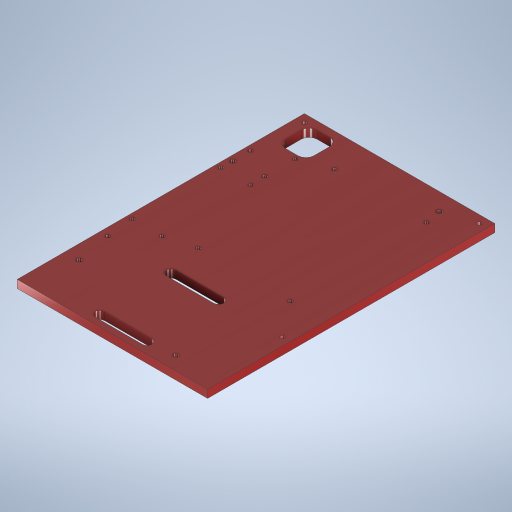
# Autodesk Inventor part: tamiya_chassis
Saved by Autodesk Inventor 2024 (Build 280153000, 153)
## iProperties
Created: 2024-01-24
Part Number: tamiya_chassis
Material: Generic
Document SubType Name: Modeling
Designer: critt
Density: 1 g/cm^3
Appearance: Default
Author: critt
## iProperties of the stored document tamiya_chassis_3DPrint.ipt
Created: 2024-01-26
Part Number: tamiya_chassis_3DPrint
Material: Generic
Document SubType Name: Modeling
Designer: critt
Density: 1 g/cm^3
Appearance: Default
Author: critt
Autodesk Inventor part; units mm, degrees
ref_plane "YZ Plane" through (0, 0, 0) normal (1, 0, 0) x (0, 1, 0)
ref_plane "XZ Plane" through (0, 0, 0) normal (0, 1, 0) x (-1, 0, 0)
ref_plane "XY Plane" through (0, 0, 0) normal (0, 0, 1) x (1, 0, 0)
sketch "Sketch1" plane through (0, 0, 0) normal (0, 1, 0) x (-1, 0, 0)
  line L0 (35.3225, -111.2173) -> (35.3225, -99.2173)
  arc A0 (39.3225, -95.2173) -> (35.3225, -99.2173) centre (39.3225, -99.2173) ccw
  line L1 (39.3225, -95.2173) -> (50.3225, -95.2173)
  line L2 (50.3225, -95.2173) -> (50.3225, -19.2173)
  line L3 (50.3225, -19.2173) -> (41.3225, -10.2173)
  line L4 (41.3225, -10.2173) -> (41.3225, 19.7827)
  line L5 (41.3225, 19.7827) -> (50.3225, 29.7827)
  line L6 (50.3225, 29.7827) -> (50.3225, 56.7827)
  line L7 (50.3225, 56.7827) -> (41.3225, 61.4627)
  line L8 (41.3225, 61.4627) -> (25.3225, 69.7827)
  line L9 (25.3225, 69.7827) -> (-44.6775, 69.7827)
  line L10 (-44.6775, 69.7827) -> (-69.6775, 56.7827)
  line L11 (-69.6775, 56.7827) -> (-69.6775, -95.2173)
  line L12 (-69.6775, -95.2173) -> (-58.6775, -95.2173)
  arc A1 (-54.6775, -99.2173) -> (-58.6775, -95.2173) centre (-58.6775, -99.2173) ccw
  line L13 (-54.6775, -99.2173) -> (-54.6775, -111.2173)
  line L14 (-54.6775, -111.2173) -> (35.3225, -111.2173)
  circle A2 centre (-1.2775, -73.2173) radius 1.6
  circle A3 centre (46.8225, -62.6173) radius 1.6
  circle A4 centre (-45.6543, -100.153) radius 1.6
  circle A5 centre (-41.1775, 61.2827) radius 1.6
  circle A6 centre (41.3225, 39.7827) radius 1.6
  circle A7 centre (46.8225, -72.6173) radius 1.6
  line L15 (-24.6775, 65.7827) -> (5.3225, 65.7827)
  arc A8 (5.3225, 59.7827) -> (5.3225, 65.7827) centre (5.3225, 62.7827) ccw
  line L16 (5.3225, 59.7827) -> (-24.6775, 59.7827)
  arc A9 (-24.6775, 65.7827) -> (-24.6775, 59.7827) centre (-24.6775, 62.7827) ccw
  line L17 (5.3225, 14.6811) -> (-24.6775, 14.6811)
  arc A10 (-24.6775, 20.8843) -> (-24.6775, 14.6811) centre (-24.6775, 17.7827) ccw
  line L18 (-24.6775, 20.8843) -> (5.3225, 20.8843)
  arc A11 (5.3225, 14.6811) -> (5.3225, 20.8843) centre (5.3225, 17.7827) ccw
  circle A12 centre (20.3225, 49.7827) radius 1.6
  circle A13 centre (20.3225, -90.2173) radius 1.6
  circle A14 centre (-39.6775, 49.7827) radius 1.6
  circle A15 centre (-39.6775, -90.2173) radius 1.6
  line L19 (25.3225, 69.7827) -> (50.3225, 69.7827)
  line L20 (50.3225, 69.7827) -> (50.3225, 56.7827)
  line L21 (-44.6775, 69.7827) -> (-69.6775, 69.7827)
  line L22 (-69.6775, 69.7827) -> (-69.6775, 56.7827)
  constraints: 46 end point, 16 centre point, 12 point on circle, 9 horizontal, 6 vertical, 1 perpendicular, 1 point on line, 62 other
extrude "Extrusion1" add sketch "Sketch1" along normal blind 5 contours L14 L13 A1 L12 L11 L10 L9 L8 L7 L6 L5 L4 L3 L2 L1 A0 L0 | L22 L21 L10 | L19 L20 L7 L8 | A2 | A7 | A12 | A13 | A14 | A15
sketch "Sketch18" plane through (0, 5, 0) normal (0, 1, 0) x (1, 0, 0)
  line L0 (-50.3225, 95.2173) -> (-50.3225, 19.2173) projected
  line L1 (-50.3225, 19.2173) -> (-41.3225, 10.2173) projected
  line L2 (-41.3225, 10.2173) -> (-41.3225, -19.7827) projected
  line L3 (-41.3225, -19.7827) -> (-50.3225, -29.7827) projected
  line L4 (-50.3225, -29.7827) -> (-50.3225, -69.7827) projected
  line L5 (-50.3225, -69.7827) -> (69.6775, -69.7827) projected
  line L6 (69.6775, -69.7827) -> (69.6775, 95.2173) projected
  line L7 (69.6775, 95.2173) -> (58.6775, 95.2173) projected
  arc A0 (54.6775, 99.2173) -> (58.6775, 95.2173) centre (58.6775, 99.2173) ccw projected
  line L8 (54.6775, 99.2173) -> (54.6775, 111.2173) projected
  line L9 (54.6775, 111.2173) -> (-35.3225, 111.2173) projected
  line L10 (-35.3225, 111.2173) -> (-35.3225, 99.2173) projected
  arc A1 (-39.3225, 95.2173) -> (-35.3225, 99.2173) centre (-39.3225, 99.2173) ccw projected
  line L11 (-39.3225, 95.2173) -> (-50.3225, 95.2173) projected
  circle A2 centre (-46.8225, 62.6173) radius 1.6 projected
  circle A3 centre (-41.3225, -39.7827) radius 1.6 projected
  circle A4 centre (45.6543, 100.153) radius 1.6 projected
  circle A5 centre (41.1775, -61.2827) radius 1.6 projected
  line L12 (-5.3225, -59.7827) -> (24.6775, -59.7827) projected
  arc A6 (24.6775, -65.7827) -> (24.6775, -59.7827) centre (24.6775, -62.7827) ccw projected
  line L13 (24.6775, -65.7827) -> (-5.3225, -65.7827) projected
  arc A7 (-5.3225, -59.7827) -> (-5.3225, -65.7827) centre (-5.3225, -62.7827) ccw projected
  line L14 (-5.3225, -14.6811) -> (24.6775, -14.6811) projected
  arc A8 (24.6775, -20.8843) -> (24.6775, -14.6811) centre (24.6775, -17.7827) ccw projected
  line L15 (24.6775, -20.8843) -> (-5.3225, -20.8843) projected
  arc A9 (-5.3225, -14.6811) -> (-5.3225, -20.8843) centre (-5.3225, -17.7827) ccw projected
  line L16 (-50.3225, 95.2173) -> (-50.3225, 111.2173)
  line L17 (-50.3225, 111.2173) -> (-35.3225, 111.2173)
  line L18 (54.6775, 111.2173) -> (69.6775, 111.2173)
  line L19 (69.6775, 111.2173) -> (69.6775, 95.2173)
  line L20 (-50.3225, 19.2173) -> (-50.3225, -29.7827)
  point P0 (0, 0)
  constraints: 10 end point, 2 perpendicular, 2 vertical, 1 point on line
extrude "Extrusion14" add sketch "Sketch18" against normal blind 5 contours L16 L17 L10 A1 L11 | L1 L2 L3 L20 | L18 L19 L7 A0 L8
sketch "Sketch20" plane through (0, 0, 0) normal (0, -1, 0) x (1, 0, 0)
  line L0 (-23.2225, 2.6207) -> (-42.0225, 2.6207) construction
  line L1 (-42.0225, 2.6207) -> (-42.0225, -53.2793) construction
  line L2 (-42.0225, -53.2793) -> (-23.2225, -53.2793) construction
  line L3 (-23.2225, -53.2793) -> (-23.2225, 2.6207) construction
  line L4 (47.6775, -4.2173) -> (-10.3225, -4.2173) construction
  line L5 (-10.3225, -4.2173) -> (-10.3225, -90.2173) construction
  line L6 (-10.3225, -90.2173) -> (47.6775, -90.2173) construction
  line L7 (47.6775, -90.2173) -> (47.6775, -4.2173) construction
  line L8 (-23.4785, -64.3733) -> (-42.5285, -64.3733) construction
  line L9 (-42.5285, -64.3733) -> (-42.5285, -83.4233) construction
  line L10 (-42.5285, -83.4233) -> (-23.4785, -83.4233) construction
  line L11 (-23.4785, -83.4233) -> (-23.4785, -64.3733) construction
  circle A0 centre (-23.2225, 2.6207) radius 1.3
  circle A1 centre (-23.2225, -53.2793) radius 1.3
  circle A2 centre (-42.0225, 2.6207) radius 1.3
  circle A3 centre (-42.0225, -53.2793) radius 1.3
  circle A4 centre (-23.4785, -64.3733) radius 1.3
  circle A5 centre (-23.4785, -83.4233) radius 1.3
  line L12 (-20.6845, -61.5793) -> (-45.3225, -61.5793) construction
  line L13 (-45.3225, -61.5793) -> (-45.3225, -86.2173) construction
  line L14 (-37.3225, -86.2173) -> (-20.6845, -86.2173) construction
  line L15 (-20.6845, -86.2173) -> (-20.6845, -61.5793) construction
  line L16 (-19.9225, 5.9207) -> (-45.3225, 5.9207) construction
  line L17 (-45.3225, 5.9207) -> (-45.3225, -56.5793) construction
  line L18 (-45.3225, -56.5793) -> (-19.9225, -56.5793) construction
  line L19 (-19.9225, -56.5793) -> (-19.9225, 5.9207) construction
  circle A6 centre (47.6775, -4.2173) radius 1.3
  circle A7 centre (-10.3225, -4.2173) radius 1.3
  circle A8 centre (-10.3225, -90.2173) radius 1.3
  circle A9 centre (47.6775, -90.2173) radius 1.3
  line L20 (64.6775, 5.7827) -> (-14.3225, 5.7827) construction
  line L21 (-14.3225, 5.7827) -> (-14.3225, -94.2173) construction
  line L22 (-14.3225, -94.2173) -> (64.6775, -94.2173) construction
  line L23 (64.6775, -94.2173) -> (64.6775, 5.7827) construction
  line L24 (64.6775, 17.7827) -> (-45.3225, 17.7827) construction
  line L25 (-45.3225, 17.7827) -> (-45.3225, -106.2173) construction
  line L26 (-37.3225, -106.2173) -> (64.6775, -106.2173) construction
  line L27 (64.6775, -106.2173) -> (64.6775, 17.7827) construction
  circle A10 centre (64.6775, 17.7827) radius 1.3
  circle A11 centre (-45.3225, 17.7827) radius 1.3
  circle A12 centre (-45.3225, -106.2173) radius 1.3
  circle A13 centre (64.6775, -106.2173) radius 1.3
  line L28 (-50.3225, -111.2173) -> (69.6775, -111.2173) construction
  line L29 (69.6775, 69.7827) -> (69.6775, -111.2173) construction
  line L30 (-50.3225, -111.2173) -> (-50.3225, 69.7827) construction
  line L31 (25.1775, 5.7827) -> (64.6775, 17.7827) construction
  line L32 (25.1775, -94.2173) -> (64.6775, -106.2173) construction
  line L33 (-42.3225, -86.2173) -> (-22.3225, -86.2173)
  line L34 (-17.3225, -91.2173) -> (-17.3225, -101.2173)
  line L35 (-22.3225, -106.2173) -> (-42.3225, -106.2173)
  line L36 (-42.3225, -101.2173) -> (-42.3225, -91.2173)
  arc A14 (-17.3225, -91.2173) -> (-22.3225, -86.2173) centre (-22.3225, -91.2173) ccw
  arc A15 (-22.3225, -106.2173) -> (-17.3225, -101.2173) centre (-22.3225, -101.2173) ccw
  arc A16 (-42.3225, -101.2173) -> (-37.3225, -106.2173) centre (-37.3225, -101.2173) ccw
  arc A17 (-37.3225, -86.2173) -> (-42.3225, -91.2173) centre (-37.3225, -91.2173) ccw
  circle A18 centre (-42.5285, -73.8983) radius 1.3
  point P0 (0, 0)
  point P1 (-32.6225, -56.5793)
  point P2 (-17.3225, -106.2173)
  dimension "d122" = 2.6
  dimension "d123" = 2.6
  dimension "d124" = 2.6
  dimension "d125" = 2.6
  dimension "d126" = 2.6
  dimension "d128" = 2.6
  dimension "d130" = 19.05
  dimension "d131" = 2.794
  dimension "d132" = 2.794
  dimension "d133" = 2.794
  dimension "d134" = 55.9
  dimension "d135" = 18.8
  dimension "d136" = 3.3
  dimension "d137" = 3.3
  dimension "d138" = 3.3
  dimension "d139" = 2.6
  dimension "d140" = 2.6
  dimension "d141" = 2.6
  dimension "d142" = 2.6
  dimension "d143" = 86
  dimension "d144" = 58
  dimension "d145" = 10
  dimension "d146" = 4
  dimension "d147" = 17
  dimension "d148" = 4
  dimension "d149" = 2.6
  dimension "d150" = 2.6
  dimension "d151" = 2.6
  dimension "d152" = 2.6
  dimension "d153" = 5
  dimension "d154" = 5
  dimension "d155" = 5
  dimension "d156" = 124
  dimension "d158" = 3.3
  dimension "d159" = 21.844
  dimension "d160" = 25
  dimension "d161" = 5
  dimension "d164" = 3
  dimension "d165" = 3
  dimension "d167" = 5
  dimension "d168" = 2.794
  dimension "d169" = 2.6
  constraints: 68 end point, 19 centre point, 16 parallel, 14 coincident, 8 horizontal, 8 perpendicular, 8 point on circle, 8 point on line, 8 tangent, 4 midpoint, 3 collinear, 3 equal radius, 1 equal length
  measures "d122" diameter of A0
  measures "d123" diameter of A1
  measures "d124" diameter of A2
  measures "d125" diameter of A3
  measures "d126" diameter of A4
  measures "d128" diameter of A5
  measures "d130" distance of L10.end L8.start
  measures "d131" distance between parallel lines of L14 L10
  measures "d132" distance between parallel lines of L15 L11
  measures "d133" distance between parallel lines of L12 L8
  measures "d134" distance of L2.end L0.start
  measures "d135" distance of L0.start L0.end
  measures "d136" distance between parallel lines of L19 L3
  measures "d137" distance between parallel lines of L16 L0
  measures "d138" distance between parallel lines of L18 L2
  measures "d139" diameter of A6
  measures "d140" diameter of A7
  measures "d141" diameter of A8
  measures "d142" diameter of A9
  measures "d143" distance of L6.end L4.start
  measures "d144" distance of L5.end L6.end
  measures "d145" distance between parallel lines of L20 L4
  measures "d146" distance between parallel lines of L5 L21
  measures "d147" distance between parallel lines of L23 L7
  measures "d148" distance between parallel lines of L22 L6
  measures "d149" diameter of A10
  measures "d150" diameter of A11
  measures "d151" diameter of A12
  measures "d152" diameter of A13
  measures "d153" distance between parallel lines of L28 L26
  measures "d154" distance between parallel lines of L29 L27
  measures "d155" distance between parallel lines of L30 L25
  measures "d156" distance of L24.end L25.end
  measures "d158" distance between parallel lines of L1 L17
  measures "d159" distance from line of L13 A4.centre
  measures "d160" distance between parallel lines of L28 L14
  measures "d161" distance from line of point (-32.623, -56.579) L12
  measures "d164" distance between parallel lines of L36 L25
  measures "d165" distance between parallel lines of L21 L34
  measures "d167" radius of A14
  measures "d168" distance between parallel lines of L25 L9
  measures "d169" diameter of A18
extrude "Extrusion15" cut sketch "Sketch20" against normal blind 10
sketch "Sketch22" plane through (0, 0, 0) normal (0, -1, 0) x (1, 0, 0)
  circle A0 centre (64.6775, -106.2173) radius 1.3 projected
  circle A1 centre (47.6775, -90.2173) radius 1.3 projected
  circle A2 centre (64.6775, 17.7827) radius 1.3 projected
  circle A3 centre (-45.3225, -106.2173) radius 1.3 projected
  circle A4 centre (-23.2225, -53.2793) radius 1.3 projected
  circle A5 centre (-42.0225, -53.2793) radius 1.3 projected
  circle A6 centre (-10.3225, -4.2173) radius 1.3 projected
  circle A7 centre (-42.5285, -73.8983) radius 1.3 projected
  circle A8 centre (-10.3225, -90.2173) radius 1.3 projected
  circle A9 centre (-23.4785, -83.4233) radius 1.3 projected
  circle A10 centre (-42.0225, 2.6207) radius 1.3 projected
  circle A11 centre (-23.2225, 2.6207) radius 1.3 projected
  circle A12 centre (-45.3225, 17.7827) radius 1.3 projected
  circle A13 centre (-23.4785, -64.3733) radius 1.3 projected
  circle A14 centre (47.6775, -4.2173) radius 1.3 projected
  arc A15 (-37.3225, -86.2173) -> (-42.3225, -91.2173) centre (-37.3225, -91.2173) ccw projected
  line L0 (-37.3225, -86.2173) -> (-22.3225, -86.2173) projected
  arc A16 (-17.3225, -91.2173) -> (-22.3225, -86.2173) centre (-22.3225, -91.2173) ccw projected
  line L1 (-17.3225, -91.2173) -> (-17.3225, -101.2173) projected
  arc A17 (-22.3225, -106.2173) -> (-17.3225, -101.2173) centre (-22.3225, -101.2173) ccw projected
  line L2 (-22.3225, -106.2173) -> (-37.3225, -106.2173) projected
  arc A18 (-42.3225, -101.2173) -> (-37.3225, -106.2173) centre (-37.3225, -101.2173) ccw projected
  line L3 (-42.3225, -101.2173) -> (-42.3225, -91.2173) projected
  line L4 (-50.3225, -111.2173) -> (-50.3225, 69.7827) projected
  line L5 (-50.3225, -111.2173) -> (69.6775, -111.2173) projected
  line L6 (69.6775, 69.7827) -> (69.6775, -111.2173) projected
  line L7 (-50.3225, 69.7827) -> (69.6775, 69.7827) projected
  circle A19 centre (-46.8225, -62.6173) radius 1.6 projected
  circle A20 centre (-41.3225, 39.7827) radius 1.6 projected
  circle A21 centre (45.6543, -100.153) radius 1.6 projected
  circle A22 centre (41.1775, 61.2827) radius 1.6 projected
  line L8 (-5.3225, 59.7827) -> (24.6775, 59.7827) projected
  arc A23 (-5.3225, 65.7827) -> (-5.3225, 59.7827) centre (-5.3225, 62.7827) ccw projected
  line L9 (24.6775, 65.7827) -> (-5.3225, 65.7827) projected
  arc A24 (24.6775, 59.7827) -> (24.6775, 65.7827) centre (24.6775, 62.7827) ccw projected
  line L10 (-5.3225, 14.6811) -> (24.6775, 14.6811) projected
  arc A25 (-5.3225, 20.8843) -> (-5.3225, 14.6811) centre (-5.3225, 17.7827) ccw projected
  line L11 (24.6775, 20.8843) -> (-5.3225, 20.8843) projected
  arc A26 (24.6775, 14.6811) -> (24.6775, 20.8843) centre (24.6775, 17.7827) ccw projected
  point P0 (0, 0)
extrude "Extrusion16" add sketch "Sketch22" against normal blind 5 contours A4 | A5 | A7 | A9 | A10 | A11 | A13
sketch "Sketch23" plane through (0, 0, 0) normal (0, -1, 0) x (1, 0, 0)
  circle A0 centre (-47.0225, 0.6207) radius 1.25 projected
  circle A1 centre (-28.2225, 0.6207) radius 1.25 projected
  circle A2 centre (-47.0225, -55.2793) radius 1.25 projected
  circle A3 centre (-28.2225, -55.2793) radius 1.25 projected
  circle A4 centre (-28.4785, -83.4233) radius 1.0922 projected
  circle A5 centre (-28.4785, -64.3733) radius 1.0922 projected
  point P0 (0, 0)
extrude "Extrusion17" cut sketch "Sketch23" against normal blind 5
sketch "Sketch24" plane through (0, 0, 0) normal (0, -1, 0) x (1, 0, 0)
  circle A0 centre (-28.2225, -55.2793) radius 1.25 projected
  circle A1 centre (-28.4785, -83.4233) radius 1.0922 projected
  circle A2 centre (-28.2225, 0.6207) radius 1.25 projected
  circle A3 centre (-47.0225, -55.2793) radius 1.25 projected
  circle A4 centre (-28.4785, -64.3733) radius 1.0922 projected
  circle A5 centre (-47.0225, 0.6207) radius 1.25 projected
  circle A6 centre (64.6775, -106.2173) radius 1.3 projected
  circle A7 centre (47.6775, -90.2173) radius 1.3 projected
  circle A8 centre (64.6775, 17.7827) radius 1.3 projected
  circle A9 centre (-45.3225, -106.2173) radius 1.3 projected
  circle A10 centre (-10.3225, -4.2173) radius 1.3 projected
  circle A11 centre (-10.3225, -90.2173) radius 1.3 projected
  circle A12 centre (-45.3225, 17.7827) radius 1.3 projected
  circle A13 centre (47.6775, -4.2173) radius 1.3 projected
  arc A14 (-37.3225, -86.2173) -> (-42.3225, -91.2173) centre (-37.3225, -91.2173) ccw projected
  line L0 (-37.3225, -86.2173) -> (-22.3225, -86.2173) projected
  arc A15 (-17.3225, -91.2173) -> (-22.3225, -86.2173) centre (-22.3225, -91.2173) ccw projected
  line L1 (-17.3225, -91.2173) -> (-17.3225, -101.2173) projected
  arc A16 (-22.3225, -106.2173) -> (-17.3225, -101.2173) centre (-22.3225, -101.2173) ccw projected
  line L2 (-22.3225, -106.2173) -> (-37.3225, -106.2173) projected
  arc A17 (-42.3225, -101.2173) -> (-37.3225, -106.2173) centre (-37.3225, -101.2173) ccw projected
  line L3 (-42.3225, -101.2173) -> (-42.3225, -91.2173) projected
  line L4 (-50.3225, -111.2173) -> (-50.3225, 69.7827) projected
  line L5 (-50.3225, -111.2173) -> (69.6775, -111.2173) projected
  line L6 (69.6775, 69.7827) -> (69.6775, -111.2173) projected
  line L7 (-50.3225, 69.7827) -> (69.6775, 69.7827) projected
  circle A18 centre (-46.8225, -62.6173) radius 1.6 projected
  circle A19 centre (-41.3225, 39.7827) radius 1.6 projected
  circle A20 centre (45.6543, -100.153) radius 1.6 projected
  circle A21 centre (41.1775, 61.2827) radius 1.6 projected
  line L8 (-5.3225, 59.7827) -> (24.6775, 59.7827) projected
  arc A22 (-5.3225, 65.7827) -> (-5.3225, 59.7827) centre (-5.3225, 62.7827) ccw projected
  line L9 (24.6775, 65.7827) -> (-5.3225, 65.7827) projected
  arc A23 (24.6775, 59.7827) -> (24.6775, 65.7827) centre (24.6775, 62.7827) ccw projected
  line L10 (-5.3225, 14.6811) -> (24.6775, 14.6811) projected
  arc A24 (-5.3225, 20.8843) -> (-5.3225, 14.6811) centre (-5.3225, 17.7827) ccw projected
  line L11 (24.6775, 20.8843) -> (-5.3225, 20.8843) projected
  arc A25 (24.6775, 14.6811) -> (24.6775, 20.8843) centre (24.6775, 17.7827) ccw projected
  circle A26 centre (-28.2225, 0.6207) radius 1.3
  circle A27 centre (-47.0225, 0.6207) radius 1.3
  circle A28 centre (-47.0225, -55.2793) radius 1.3
  circle A29 centre (-28.2225, -55.2793) radius 1.3
  circle A30 centre (-28.4785, -83.4233) radius 1.3
  circle A31 centre (-28.4785, -64.3733) radius 1.3
  circle A32 centre (-47.0225, -73.8983) radius 1.3
  line L12 (-47.0225, -55.2793) -> (-47.0225, -73.8983) construction
  line L13 (-47.0225, -73.8983) -> (-28.4785, -64.3733) construction
  line L14 (-47.0225, -73.8983) -> (-28.4785, -83.4233) construction
  point P0 (0, 0)
  dimension "d174" = 2.6
  constraints: 7 centre point, 6 coincident, 6 end point, 6 equal radius, 1 equal length, 1 vertical
  measures "d174" diameter of A30
extrude "Extrusion18" cut sketch "Sketch24" against normal blind 5 contours A2 | A5 | A26 | A27 | A28 | A29 | A30 | A31 | A32
sketch "Sketch25" plane through (0, 0, 0) normal (0, -1, 0) x (1, 0, 0)
  circle A0 centre (-28.2225, -55.2793) radius 1.3 projected
  circle A1 centre (-28.4785, -64.3733) radius 1.3 projected
  circle A2 centre (-47.0225, -55.2793) radius 1.3 projected
  circle A3 centre (-47.0225, 0.6207) radius 1.3 projected
  circle A4 centre (-28.4785, -83.4233) radius 1.3 projected
  circle A5 centre (-47.0225, -73.8983) radius 1.3 projected
  circle A6 centre (-28.2225, 0.6207) radius 1.3 projected
  circle A7 centre (64.6775, -106.2173) radius 1.3 projected
  circle A8 centre (47.6775, -90.2173) radius 1.3 projected
  circle A9 centre (64.6775, 17.7827) radius 1.3 projected
  circle A10 centre (-45.3225, -106.2173) radius 1.3 projected
  circle A11 centre (-10.3225, -4.2173) radius 1.3 projected
  circle A12 centre (-10.3225, -90.2173) radius 1.3 projected
  circle A13 centre (-45.3225, 17.7827) radius 1.3 projected
  circle A14 centre (47.6775, -4.2173) radius 1.3 projected
  arc A15 (-37.3225, -86.2173) -> (-42.3225, -91.2173) centre (-37.3225, -91.2173) ccw projected
  line L0 (-37.3225, -86.2173) -> (-22.3225, -86.2173) projected
  arc A16 (-17.3225, -91.2173) -> (-22.3225, -86.2173) centre (-22.3225, -91.2173) ccw projected
  line L1 (-17.3225, -91.2173) -> (-17.3225, -101.2173) projected
  arc A17 (-22.3225, -106.2173) -> (-17.3225, -101.2173) centre (-22.3225, -101.2173) ccw projected
  line L2 (-22.3225, -106.2173) -> (-37.3225, -106.2173) projected
  arc A18 (-42.3225, -101.2173) -> (-37.3225, -106.2173) centre (-37.3225, -101.2173) ccw projected
  line L3 (-42.3225, -101.2173) -> (-42.3225, -91.2173) projected
  line L4 (-50.3225, -111.2173) -> (-50.3225, 69.7827) projected
  line L5 (-50.3225, -111.2173) -> (69.6775, -111.2173) projected
  line L6 (69.6775, 69.7827) -> (69.6775, -111.2173) projected
  line L7 (-50.3225, 69.7827) -> (69.6775, 69.7827) projected
  circle A19 centre (-46.8225, -62.6173) radius 1.6 projected
  circle A20 centre (-41.3225, 39.7827) radius 1.6 projected
  circle A21 centre (45.6543, -100.153) radius 1.6 projected
  circle A22 centre (41.1775, 61.2827) radius 1.6 projected
  line L8 (-5.3225, 59.7827) -> (24.6775, 59.7827) projected
  arc A23 (-5.3225, 65.7827) -> (-5.3225, 59.7827) centre (-5.3225, 62.7827) ccw projected
  line L9 (24.6775, 65.7827) -> (-5.3225, 65.7827) projected
  arc A24 (24.6775, 59.7827) -> (24.6775, 65.7827) centre (24.6775, 62.7827) ccw projected
  line L10 (-5.3225, 14.6811) -> (24.6775, 14.6811) projected
  arc A25 (-5.3225, 20.8843) -> (-5.3225, 14.6811) centre (-5.3225, 17.7827) ccw projected
  line L11 (24.6775, 20.8843) -> (-5.3225, 20.8843) projected
  arc A26 (24.6775, 14.6811) -> (24.6775, 20.8843) centre (24.6775, 17.7827) ccw projected
  line L12 (-17.3225, -86.2173) -> (-24.3225, -86.2173)
  line L13 (-24.3225, -86.2173) -> (-24.3225, -106.2173)
  line L14 (-24.3225, -106.2173) -> (-17.3225, -106.2173)
  line L15 (-17.3225, -106.2173) -> (-17.3225, -86.2173)
  line L16 (-37.3225, -86.2173) -> (-22.3225, -86.2173) projected
  point P0 (0, 0)
  dimension "d179" = 26
  constraints: 8 end point, 3 collinear, 2 parallel, 1 horizontal, 1 perpendicular
  measures "d179" distance between parallel lines of L4 L13
extrude "Extrusion20" add sketch "Sketch25" against normal blind 5 contours L0 A16 L1 A17 L2 L13
fillet "Fillet2" radius 5 2 edges at (-24.3225, 2.5, -86.2173) (-24.3225, 2.5, -106.2173)
body "Solid1"
